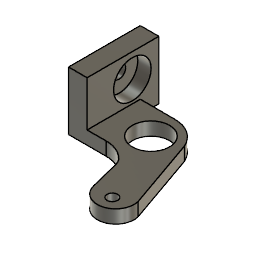
ACOPLE_RUEDA_BARRA_DER (Autodesk Fusion 360 design; units mm, degrees)
Autodesk Fusion 360 part; units mm, degrees
note: some values were not read from the file. Chosen so that the rebuilt part matches the saved one: which bodies a step acts on.
sketch "Boceto2" plane through (0, 0, 0) normal (0, 0, 1) x (1, 0, 0)
  arc A0 (9.5071, 3.1073) -> (-1.0383, 10) centre (-1.0383, -1.5134) ccw
  line L0 (-14, -10) -> (-14, 17)
  line L1 (-14, 10) -> (-1.0383, 10)
  arc A1 (1.2721, -13.3803) -> (-6.8217, -10) centre (-6.8217, -21.38) ccw
  line L2 (5.4387, -27.1021) -> (18.8818, -23.7213) construction
  line L3 (12.6785, -27.1892) -> (14, -27.1892) construction
  line L4 (-14, 17) -> (-21, 17)
  arc A2 (5.4387, -27.1021) -> (18.8818, -23.7213) centre (12.1602, -25.4117) ccw
  circle A3 centre (0, 0) radius 2.5
  circle A4 centre (12.6785, -27.1892) radius 2
  line L5 (-21, -10) -> (-14, -10)
  line L6 (-6.8217, -10) -> (-14, -10)
  line L7 (-21, 17) -> (-21, -10)
  line L8 (0, 0) -> (12.6785, -27.1892) construction
  circle A5 centre (0, 0) radius 7
  arc A6 (2.5649, -15.6756) -> (1.2721, -13.3803) centre (-2.2841, -16.8951) ccw
  line L9 (2.5649, -15.6756) -> (5.4387, -27.1021)
  line L10 (-21, 17) -> (-21, -10)
  line L11 (18.8818, -23.7213) -> (9.5071, 3.1073)
  dimension "d85" = 5
  dimension "d86" = 14
  dimension "d87" = 4
  dimension "d88" = 30
  dimension "d89" = 65
  dimension "d90" = 10
  dimension "d91" = 10
  dimension "d92" = 7
  dimension "d93" = 14
  dimension "d94" = 5
  dimension "d95" = 7
  dimension "d96" = 10
  dimension "d97" = 7
  dimension "d98" = 27
  constraint coincident A3.centre L8.start
  constraint concentric A3 A5
  constraint coincident L3.start A4.centre
  constraint horizontal L3
  constraint horizontal L1
  constraint horizontal L6
  constraint vertical L0
  constraint coincident L1.start L0
  constraint tangent A1 L6
  constraint tangent A1 A6
  constraint tangent A6 L9
  constraint perpendicular L0 L4
  constraint perpendicular L4 L10
  constraint tangent A0 L1
  constraint perpendicular L2 L9
  constraint tangent A2 L9
  measures "d85" diameter of A3
  measures "d86" diameter of A5
  measures "d87" diameter of A4
  measures "d88" distance of L3.start A3.centre
  measures "d89" angle of L3 L8
  measures "d90" distance of A3.centre L1
  measures "d91" distance of A3.centre L11
  measures "d92" distance of L3.start L11
  measures "d93" distance of A3.centre L0
  measures "d94" radius of A6
  measures "d95" distance of L3.start L9
  measures "d96" distance of A3.centre L6
  measures "d97" distance of L0 L10
  measures "d98" distance of L4 L5
sketch "Boceto4" plane through (-21, 0, 0) normal (-1, 0, 0) x (0, -1, 0)
  line L0 (-17, 0) -> (10, 0)
  line L1 (10, 0) -> (10, 22)
  line L2 (10, 22) -> (-17, 22)
  line L3 (-17, 22) -> (-17, 0)
  circle A0 centre (-7, 13) radius 7.05
  circle A1 centre (-7, 13) radius 2.5
  dimension "d52" = 14.1
  dimension "d53" = 5
  dimension "d54" = 10
  dimension "d55" = 9
  constraint concentric A0 A1
  measures "d52" diameter of A0
  measures "d53" diameter of A1
  measures "d54" distance of L3 A0.centre
  measures "d55" distance of L2 A0.centre
extrude "Extruir18" add sketch "Boceto2" along normal blind 5 contours A0 L0 L1 A1 A2 L6 A6 L9 L11 makes body 1
extrude "Extruir19" add sketch "Boceto2" along normal blind 22 contours L0 L4 L5 L7 L10 bodies 1
extrude "Extruir20" cut sketch "Boceto4" against normal blind 24 contours A0 bodies 1 makes body 2 at (-14, 0, 0)
extrude "Extruir21" cut sketch "Boceto4" against normal blind 15 contours A1 bodies 1 2
extrude "Extruir22" cut sketch "Boceto4" along normal blind 2 contours L0 L1 L2 L3 bodies 2
extrude "Extruir23" add sketch "Boceto4" against normal blind 2 contours A0 bodies 1 2
extrude "Extruir3" [suppressed]
extrude "Extruir4" [suppressed]
extrude "Extruir5" [suppressed]
sketch "Boceto3" plane through (-21, 0, 0) normal (-1, 0, 0) x (0, -1, 0)
  line L0 (-17, 0) -> (10, 0)
  line L1 (10, 0) -> (10, 20)
  line L2 (10, 20) -> (-17, 20)
  line L3 (-17, 20) -> (-17, 0)
  circle A0 centre (-7, 10) radius 7
  circle A1 centre (-7, 10) radius 2.5
  dimension "d38" = 14
  dimension "d39" = 10
  dimension "d40" = 10
  dimension "d41" = 5
  constraint concentric A0 A1
  measures "d38" diameter of A0
  measures "d39" distance of L3 A0.centre
  measures "d40" distance of L2 A0.centre
  measures "d41" diameter of A1
extrude "Extruir6" [suppressed]
extrude "Extruir7" [suppressed]
